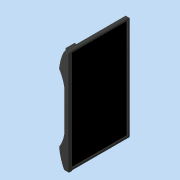
# Autodesk Inventor part: DellP2317H
Saved by Autodesk Inventor 2017 (Build 210142000, 142)
## iProperties
Created: 2018-10-04
Part Number: DellP2317H
Material: ABS Plastic
Document SubType Name: Modeling
Designer: mailb
Density: 1.06 g/cm^3
Appearance: Smooth - Black
Author: mailb
Autodesk Inventor part; units mm, degrees
ref_plane "YZ Plane" through (0, 0, 0) normal (1, 0, 0) x (0, 1, 0)
ref_plane "XZ Plane" through (0, 0, 0) normal (0, 1, 0) x (-1, 0, 0)
ref_plane "XY Plane" through (0, 0, 0) normal (0, 0, 1) x (1, 0, 0)
sketch "Sketch1" plane through (0, 0, 0) normal (1, 0, 0) x (0, 1, 0)
  line L0 (266.7, 158.75) -> (-266.7, 158.75)
  line L1 (-266.7, 158.75) -> (-266.7, -158.75)
  line L2 (-266.7, -158.75) -> (266.7, -158.75)
  line L3 (266.7, -158.75) -> (266.7, 158.75)
  line L4 (266.7, 158.75) -> (-266.7, -158.75) construction
  line L5 (-266.7, 158.75) -> (266.7, -158.75) construction
  point P0 (0, 0)
  dimension "d0" = 533.4
  dimension "d1" = 317.5
  constraints: 12 end point, 2 midpoint, 2 parallel, 1 horizontal, 1 perpendicular
  measures "d0" distance of L2.end L1.end
  measures "d1" distance of L1.end L0.end
extrude "Extrusion1" add sketch "Sketch1" along normal blind 20.32
sketch "Sketch2" plane through (20.32, 0, 0) normal (1, 0, 0) x (0, 0, -1)
  line L0 (-158.75, 266.7) -> (-158.75, -266.7) projected
  line L1 (158.75, 266.7) -> (-158.75, 266.7) projected
  line L2 (-158.75, -266.7) -> (-140.97, -266.7)
  line L3 (-140.97, -266.7) -> (-140.97, 266.7)
  line L4 (-140.97, 266.7) -> (-158.75, 266.7)
  line L5 (-158.75, 266.7) -> (-158.75, -266.7)
  line L6 (158.75, 266.7) -> (-140.97, 266.7)
  line L7 (-140.97, 266.7) -> (-140.97, -266.7)
  line L8 (-140.97, -266.7) -> (158.75, -266.7)
  line L9 (158.75, -266.7) -> (158.75, 266.7)
  point P0 (0, 0)
  dimension "d4" = 17.78
  constraints: 16 end point, 4 parallel, 2 horizontal, 2 perpendicular, 1 point on line
  measures "d4" distance of L4.end L3.end
extrude "Extrusion2" cut sketch "Sketch2" against normal blind 2.54 contours L1 L9 L8 L3
sketch "Sketch3" plane through (17.78, 0, 0) normal (1, 0, 0) x (0, 0, -1)
  line L0 (-140.97, -266.7) -> (-140.97, 266.7) projected
  line L1 (-140.97, 266.7) -> (-140.97, 256.54)
  line L2 (-140.97, -266.7) -> (-140.97, -256.54)
  line L3 (158.75, -266.7) -> (158.75, 266.7) projected
  line L4 (158.75, 0) -> (148.59, 0)
  line L5 (-140.97, -256.54) -> (148.59, -256.54)
  line L6 (148.59, -256.54) -> (148.59, 256.54)
  line L7 (148.59, 256.54) -> (-140.97, 256.54)
  line L8 (-140.97, 256.54) -> (-140.97, -256.54)
  point P0 (0, 0)
  dimension "d7" = 10.16
  dimension "d8" = 10.16
  dimension "d9" = 10.16
  constraints: 14 end point, 2 horizontal, 2 parallel, 2 point on line, 1 midpoint, 1 perpendicular
  measures "d7" distance of L0.end L1.end
  measures "d8" distance of L0.start L2.end
  measures "d9" distance of L4.start L4.end
extrude "Extrusion3" cut sketch "Sketch3" against normal blind 5.08
sketch "Sketch4" plane through (0, -266.7, 158.75) normal (0, 0, 1) x (1, 0, 0)
  line L0 (0, 266.7) -> (-30.48, 266.7)
  line L1 (-30.48, 266.7) -> (-30.48, 393.7)
  line L2 (-30.48, 266.7) -> (-30.48, 139.7)
  line L3 (0, 0) -> (20.32, 0) projected
  spline S0 degree 2 poles (0, 0) (-29.2196, 51.877) (-30.48, 139.7) knots 0 0 0 1 1 1
  spline S1 degree 2 poles (0, 533.4) (-29.2196, 481.523) (-30.48, 393.7) knots 0 0 0 1 1 1
  line L4 (0, 0) -> (0, 533.4)
  line L5 (20.32, 533.4) -> (20.32, 0) projected
  point P0 (-20.6375, 53.975)
  point P1 (-20.6375, 479.425)
  dimension "d12" = 30.48
  dimension "d13" = 127
  dimension "d14" = 127
  constraints: 8 end point, 2 symmetric about line, 2 vertical, 1 horizontal, 1 parallel, 6 other
  measures "d12" distance of L0.start L0.end
  measures "d13" distance of L0.end L1.end
  measures "d14" distance of L0.end L2.end
extrude "Extrusion4" add sketch "Sketch4" against normal blind 317.5
sketch "Sketch5" plane through (17.78, 266.7, 140.97) normal (0, 1, 0) x (1, 0, 0)
  line L0 (-17.78, 299.72) -> (0, 299.72) projected
  line L1 (-48.26, -17.78) -> (-48.26, 299.72) projected
  spline S0 degree 2 poles (-17.78, 299.72) (-47.3289, 249.7338) (-48.26, 184.15) knots 0 0 0 1 1 1
  line L2 (-48.26, 184.15) -> (-48.26, 299.72)
  line L3 (-48.26, 299.72) -> (-17.78, 299.72)
  point P0 (-17.78, 140.97)
  point P1 (-39.6875, 247.65)
  constraints: 4 end point, 1 collinear, 1 horizontal, 1 point on line, 3 other
extrude "Extrusion5" cut sketch "Sketch5" against normal blind 533.4
fillet "Fillet1" radius 3.81 4 edges at (8.89, 266.7, -158.75) (8.89, -266.7, -158.75) (10.16, -266.7, 158.75) (10.16, 266.7, 158.75)
fillet "Fillet2" radius 1.27 2 edges at (15.24, -256.54, -148.59) (15.24, 256.54, -148.59)
chamfer "Chamfer1" distance 1.27 angle 45 5 edges at (17.78, 256.54, -3.175) (17.78, 256.168, -148.218) (17.78, 0, -148.59) (17.78, -256.168, -148.218) (17.78, -256.54, -3.175)
sketch "Sketch6" plane through (-30.48, -127, 158.75) normal (0, 0, 1) x (1, 0, 0)
  line L0 (0, 0) -> (0, 254) projected
  line L1 (0, 127) -> (30.48, 127)
  line L2 (30.48, 127) -> (30.48, 228.6)
  line L3 (30.48, 127) -> (30.48, 25.4)
  line L4 (0, 127) -> (0, 304.8)
  line L5 (0, 127) -> (0, -50.8)
  spline S0 degree 2 poles (0, -50.8) (21.577, -20.7599) (30.48, 25.4) knots 0 0 0 1 1 1
  spline S1 degree 2 poles (0, 304.8) (21.577, 274.7599) (30.48, 228.6) knots 0 0 0 1 1 1
  point P0 (17.4625, -19.05)
  point P1 (17.4625, 273.05)
  dimension "d24" = 101.6
  dimension "d25" = 101.6
  dimension "d26" = 177.8
  dimension "d27" = 177.8
  constraints: 10 end point, 3 vertical, 1 horizontal, 1 midpoint, 1 perpendicular, 1 symmetric about line, 6 other
  measures "d24" distance of L1.end L2.end
  measures "d25" distance of L1.end L3.end
  measures "d26" distance of L1.start L4.end
  measures "d27" distance of L1.start L5.end
extrude "Extrusion6" cut sketch "Sketch6" against normal blind 78.74
fillet "Fillet3" radius 127 2 edges at (0, -101.6, 119.38) (0, 101.6, 119.38)
sketch "Sketch7" plane through (0, 266.7, 154.94) normal (0, 1, 0) x (1, 0, 0)
  line L0 (-2.0826, -3.81) -> (20.32, -3.81) projected
  line L1 (0, -3.81) -> (0, 12.7)
  line L2 (0, 12.7) -> (-10.16, 12.7)
  line L3 (-10.16, 12.7) -> (-10.16, 58.42)
  line L4 (-10.16, 58.42) -> (0, 58.42)
  line L5 (0, 58.42) -> (0, 12.7)
  point P0 (0, 154.94)
  dimension "d31" = 16.51
  dimension "d32" = 10.16
  dimension "d33" = 45.72
  constraints: 10 end point, 2 parallel, 1 horizontal, 1 perpendicular, 1 point on line
  measures "d31" distance of L1.start L1.end
  measures "d32" distance of L3.end L4.end
  measures "d33" distance of L2.end L3.end
extrude "Extrusion7" add sketch "Sketch7" against normal blind 65.7225
fillet "Fillet4" radius 25.4 1 edges at (-10.16, 245.5271, 120.309)
sketch "Sketch8" plane through (-30.48, -127, -43.18) normal (-1, 0, 0) x (0, 0, 1)
  line L0 (123.19, 214.5104) -> (123.19, 39.4896) projected
  line L1 (123.19, 127) -> (85.09, 127)
  line L2 (85.09, 127) -> (38.1, 127)
  circle A0 centre (38.1, 127) radius 46.99
  point P0 (43.18, 127)
  dimension "d37" = 38.1
  dimension "d38" = 46.99
  dimension "d39" = 93.98
  constraints: 4 end point, 1 centre point, 1 coincident, 1 horizontal, 1 midpoint, 1 point on line
  measures "d37" distance of L1.start L1.end
  measures "d38" distance of L1.end L2.end
  measures "d39" diameter of A0
extrude "Extrusion8" add sketch "Sketch8" against normal blind 7.9375
extrude "Extrusion9" add sketch "Sketch8" along normal blind 44.45
body "Solid1"
